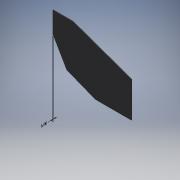
# Autodesk Inventor part: endplate
Saved by Autodesk Inventor 2018 (Build 220112000, 112)
## iProperties
Created: 2018-02-23
Part Number: endplate
Material: CFRP
Document SubType Name: Modeling
Designer: ku_sk
Density: 1.43 g/cm^3
Appearance: カーボンファイバー
Author: ku_sk
Autodesk Inventor part; units mm, degrees
ref_plane "YZ Plane" through (0, 0, 0) normal (1, 0, 0) x (0, 1, 0)
ref_plane "XZ Plane" through (0, 0, 0) normal (0, 1, 0) x (-1, 0, 0)
ref_plane "XY Plane" through (0, 0, 0) normal (0, 0, 1) x (1, 0, 0)
sketch "スケッチ1" plane through (0, 0, 0) normal (0, 1, 0) x (-1, 0, 0)
  line L0 (-300, 280) -> (300, 280)
  line L1 (300, 280) -> (300, -280)
  line L2 (300, -280) -> (-300, -280)
  line L3 (-300, -280) -> (-300, 280)
  line L4 (-300, 280) -> (300, -280) construction
  line L5 (300, 280) -> (-300, -280) construction
  point P0 (0, 0)
  dimension "d0" = 600
  dimension "d1" = 560
  constraints: 12 end point, 2 midpoint, 2 parallel, 1 horizontal, 1 perpendicular
  measures "d0" distance of L0.start L0.end
  measures "d1" distance of L2.end L0.start
extrude "押し出し1" add sketch "スケッチ1" along normal mid plane 6
sketch "スケッチ3" plane through (0, -3, 0) normal (0, -1, 0) x (1, 0, 0)
  circle A0 centre (-40, 115) radius 2.5
  line L0 (300, -280) -> (300, 280) projected
  line L1 (-300, -280) -> (300, -280) projected
  circle A1 centre (-140, 185) radius 2.5
  circle A2 centre (280, 40) radius 2.5
  point P0 (0, 0)
  dimension "d10" = 5
  dimension "d15" = 5
  dimension "d16" = 320
  dimension "d17" = 20
  dimension "d18" = 5
  dimension "d24" = 75
  dimension "d25" = 320
  dimension "d26" = 420
  dimension "d27" = 145
  constraints: 3 centre point
  measures "d10" diameter of A0
  measures "d15" diameter of A1
  measures "d16" distance from line of L1 A2.centre
  measures "d17" distance from line of L0 A2.centre
  measures "d18" diameter of A2
  measures "d24" vertical distance of A0.centre A2.centre
  measures "d25" horizontal distance of A0.centre A2.centre
  measures "d26" horizontal distance of A1.centre A2.centre
  measures "d27" vertical distance of A2.centre A1.centre
extrude "押し出し4" cut sketch "スケッチ3" against normal through all
sketch "スケッチ5" plane through (0, -3, 0) normal (0, -1, 0) x (1, 0, 0)
  line L0 (300, 250) -> (-300, 250)
  line L1 (-250, 280) -> (-250, -280) construction
  line L2 (-300, -250) -> (300, -250)
  line L3 (250, -280) -> (250, 280) construction
  line L4 (-300, 280) -> (300, 280)
  line L5 (-150, 280) -> (300, 120)
  line L6 (300, 280) -> (300, -280)
  line L7 (-300, -280) -> (-300, 280)
  line L8 (-300, 120) -> (-144.115427, -150)
  line L9 (-144.115427, -150) -> (300, -150)
  line L10 (300, -280) -> (300, 280)
  point P0 (0, 0)
  dimension "d32" = 100
  dimension "d33" = 130
  dimension "d34" = 400
  dimension "d35" = 60
  dimension "d46" = 270
  constraints: 6 end point, 4 point on line, 1 horizontal, 1 vertical alignment
  measures "d32" distance from line of L5.start L1
  measures "d33" distance from line of L0 L8.start
  measures "d34" distance between parallel lines of L0 L9
  measures "d35" angle of L9 L8
  measures "d46" distance of L9.end L5.end
sketch "スケッチ5 outline for 押し出し5" plane through (0, -3, 0) normal (0, -1, 0) x (1, 0, 0)
  line L0 (300, 120) -> (300, 280)
  line L1 (-150, 280) -> (300, 120)
  line L2 (300, 280) -> (-150, 280)
  line L3 (-300, 120) -> (-300, -280)
  line L4 (-144.115427, -150) -> (-300, 120)
  line L5 (300, -150) -> (-144.115427, -150)
  line L6 (300, -280) -> (300, -150)
  line L7 (-300, -280) -> (300, -280)
extrude "押し出し5" cut sketch "スケッチ5 outline for 押し出し5" against normal through all
chamfer "面取り2" distance 170 distance2 100 1 edges at (-144.1154, 0, -150) measured on face at (151.9615, -1, -150)
